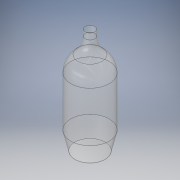
# Autodesk Inventor part: 0
Saved by Autodesk Inventor 2019 (Build 230136000, 136)
## iProperties
Company: Mechanomy LLC
Created: 2020-04-16
Part Number: 0
Material: PET Plastic
Document SubType Name: Sheet Metal
Designer: Ben
Density: 1.541 g/cm^3
Appearance: Polycarbonate - Clear
Sheet Metal Rule: Default_mm
Description: Face shield made from a 2L soda bottle
Stock Number: 0
Author: Ben
Title: SodaShield
Revision Number: 0
Autodesk Inventor part; units mm, degrees
ref_plane "YZ Plane" through (0, 0, 0) normal (1, 0, 0) x (0, 1, 0)
ref_plane "XZ Plane" through (0, 0, 0) normal (0, 1, 0) x (-1, 0, 0)
ref_plane "XY Plane" through (0, 0, 0) normal (0, 0, 1) x (1, 0, 0)
sketch "Sketch1" plane through (0, 0, 0) normal (0, 0, 1) x (1, 0, 0)
  line L0 (0, 0) -> (-13.73, 0)
  line L1 (-13.73, 0) -> (-13.73, -17)
  arc A0 (-34.11, -61.5) -> (-13.73, -17) centre (-72.5032, -17) ccw
  arc A1 (-34.11, -61.5) -> (-54.49, -106) centre (4.2832, -106) ccw
  line L2 (-54.49, -106) -> (-54.49, -246.2)
  line L3 (-54.49, -246.2) -> (-42.6683, -297)
  line L4 (-42.6683, -297) -> (0, -297)
  line L5 (0, -297) -> (0, 0)
  line L6 (0, -356.4) -> (0, 59.4) projected
  dimension "d0" = 13.73
  dimension "d1" = 17
  dimension "d2" = 54.49
  dimension "d3" = 106
  dimension "d4" = 13.1
  dimension "d5" = 297
  dimension "d6" = 50.8
  constraints: 12 end point, 4 point on circle, 3 tangent, 2 centre point, 2 horizontal, 2 perpendicular, 1 equal radius, 1 vertical
  measures "d0" distance of L0.start L0.end
  measures "d1" distance of L0.end L1.end
  measures "d2" distance from line of L0.start L2
  measures "d3" distance from line of L2.start L0
  measures "d4" angle of L2 L3
  measures "d5" distance of L4.end L0.start
  measures "d6" vertical distance of L2.end L3.end
revolve "Revolution1" add sketch "Sketch1" angle 360 about axis through (0, -10, 0) along (0, 1, 0)
shell "Shell1" thickness 0.5 removed faces 1 at (0.5517, 0, -4.0152)
sketch "Sketch2" plane through (0, 0, 0) normal (0, 0, 1) x (1, 0, 0)
  line L0 (53.99, -106) -> (-53.99, -106) projected
  line L1 (13.73, 0) -> (-13.73, 0) construction
  line L2 (-53.99, 0) -> (53.99, 0)
  line L3 (53.99, 0) -> (53.99, -46)
  line L4 (53.99, -46) -> (-53.99, -46)
  line L5 (-53.99, -46) -> (-53.99, 0)
  line L6 (53.99, -266.2) -> (-53.99, -266.2)
  line L7 (-53.99, -266.2) -> (-53.99, -297)
  line L8 (-53.99, -297) -> (53.99, -297)
  line L9 (53.99, -297) -> (53.99, -266.2)
  line L10 (42.6683, -297) -> (-42.6683, -297) projected
  line L11 (54.49, -246.2) -> (-54.49, -246.2) projected
  point P0 (0, 0)
  dimension "d10" = 60
  dimension "d11" = 20
  constraints: 16 end point, 5 parallel, 3 collinear, 2 horizontal, 2 midpoint, 2 perpendicular
  measures "d10" distance between parallel lines of L0 L4
  measures "d11" distance between parallel lines of L6 L11
sketch "Sketch3" plane through (0, 0, 0) normal (0, 0, 1) x (1, 0, 0)
  line L0 (-0.5, 0) -> (0.5, 0)
  line L1 (0.5, 0) -> (0.5, -266.2)
  line L2 (0.5, -266.2) -> (-0.5, -266.2)
  line L3 (-0.5, -266.2) -> (-0.5, 0)
  line L4 (49.8358, -266.2) -> (-49.8358, -266.2) projected
  point P0 (0, 0)
  point P1 (0, 0)
  dimension "d15" = 1
  constraints: 8 end point, 2 parallel, 1 coincident, 1 collinear, 1 horizontal, 1 midpoint, 1 perpendicular
  measures "d15" distance between parallel lines of L3 L1
sketch "Sketch4" plane through (340.0931, -246.1426, -50.8714) normal (-0.0092, 0, 1) x (1, 0, 0.0092)
  line L0 (-31, 200.1426) -> (-30, 200.1426)
  line L1 (-30, 200.1426) -> (-30, 30)
  line L2 (-30, 30) -> (-31, 30)
  line L3 (-31, 30) -> (-31, 200.1426)
  line L4 (-309.6074, 200.1426) -> (-308.6074, 200.1426)
  line L5 (-308.6074, 200.1426) -> (-308.6074, 30)
  line L6 (-308.6074, 30) -> (-309.6074, 30)
  line L7 (-309.6074, 30) -> (-309.6074, 200.1426)
  line L8 (-0.8007, 200.1426) -> (-338.8067, 200.1426) projected
  line L9 (0, 0) -> (0, 140.1426) projected
  line L10 (0, 0) -> (-339.6074, 0) projected
  line L11 (-339.6074, 140.1426) -> (-339.6074, 0) projected
  dimension "d18" = 1
  dimension "d19" = 30
  dimension "d20" = 30
  dimension "d21" = 30
  constraints: 16 end point, 4 parallel, 2 equal length, 2 horizontal, 2 perpendicular, 1 collinear, 1 point on line
  measures "d18" distance of L0.start L0.end
  measures "d19" distance between parallel lines of L9 L1
  measures "d20" distance between parallel lines of L10 L2
  measures "d21" distance between parallel lines of L11 L7
sketch "Sketch16" plane through (340.1023, -246.2, -51.3714) normal (0.0092, 0, -1) x (-1, 0, -0.0092)
  line L0 (0, 1) -> (30.0046, 31.0046)
  line L1 (30.0046, 30.0574) -> (30.0046, 140.2) projected
  line L2 (0, 140.2) -> (0, 0) projected
  point P0 (339.6166, 246.2)
  dimension "d87" = 45
  dimension "d88" = 1
  constraints: 2 end point, 2 point on line
  measures "d87" angle of L2 L0
  measures "d88" distance of L0.start L2.end
sketch "Sketch23" plane through (0.5, -246.2, -54.4877) normal (0.0092, 0, -1) x (-1, 0, -0.0092)
  line L0 (0, 1) -> (-30.0046, 31.0046)
  line L1 (0, 0) -> (0, 140.2) projected
  line L2 (-30.0046, 140.2) -> (-30.0046, 30.0574) projected
  line L3 (-339.6166, 0) -> (0, 0) projected
  point P0 (0, 246.2)
  dimension "d136" = 45
  dimension "d137" = 1
  constraints: 2 end point, 2 point on line
  measures "d136" angle of L1 L0
  measures "d137" distance from line of L3 L0.start
sketch "Sketch17" plane through (202.4892, -243.6006, -50.6341) normal (-0.0092, 0, 1) x (1, 0, 0.0092)
  line L0 (105.596, 0) -> (105.596, 30.0046)
  line L1 (105.9965, 30.0046) -> (0, 30.0046) projected
  line L2 (0, 0) -> (136.0011, 0) projected
  line L3 (106.596, 27.458) -> (106.596, 137.6006) projected
  point P0 (-202.016, 243.6006)
  dimension "d101" = 1
  constraints: 2 end point, 2 point on line, 1 vertical
  measures "d101" distance between parallel lines of L3 L0
sketch "Sketch24" plane through (2.081, -243.6006, -52.4731) normal (-0.0092, 0, 1) x (1, 0, 0.0092)
  line L0 (31.0046, 30.0046) -> (31.0046, 0)
  line L1 (-1.5994, 0) -> (136.0011, 0) projected
  line L2 (136.0011, 30.0046) -> (28.4052, 30.0046) projected
  point P0 (-1.5994, 243.6006)
  point P1 (0, 0)
  point P2 (136.0011, 0)
  point P3 (30.0046, 30.0046)
  point P4 (-1.5994, -2.5994)
  point P5 (28.4052, 27.458)
  dimension "d138" = 1
  constraints: 2 end point, 1 vertical, 4 other
  measures "d138" distance from line of point (30.005, 30.005) L0
equation "\"BendRadius\" = Thickness"
equation "\"BendReliefWidth\" = Thickness"
equation "\"BendReliefDepth\" = 0.5 * Thickness"
equation "\"CornerReliefSize\" = 4 * Thickness"
equation "\"MinimumRemnant\" = 2 * Thickness"
equation "\"TransitionRadius\" = BendRadius"
equation "\"JacobiRadiusSize\" = BendRadius"
equation "\"GapSize\" = Thickness"
equation "\"Thickness\" = 0.5"
body "Solid1"
